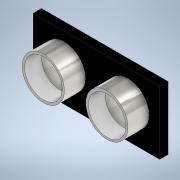
# Autodesk Inventor part: US sensor
Saved by Autodesk Inventor 2021 (Build 250183000, 183)
## iProperties
Created: 2021-07-04
Part Number: US sensor
Material: Generic
Document SubType Name: Modeling
Designer: Manojgouda K R
Density: 1 g/cm^3
Appearance: Default
Author: Manojgouda K R
Autodesk Inventor part; units mm, degrees
ref_plane "YZ Plane" through (0, 0, 0) normal (1, 0, 0) x (0, 1, 0)
ref_plane "XZ Plane" through (0, 0, 0) normal (0, 1, 0) x (-1, 0, 0)
ref_plane "XY Plane" through (0, 0, 0) normal (0, 0, 1) x (1, 0, 0)
sketch "Sketch1" plane through (0, 0, 0) normal (0, 0, 1) x (1, 0, 0)
  line L0 (-9.2175, -0.9972) -> (-3.2175, -0.9972)
  line L1 (-3.2175, -0.9972) -> (-3.2175, -3.9972)
  line L2 (-3.2175, -3.9972) -> (-9.2175, -3.9972)
  line L3 (-9.2175, -3.9972) -> (-9.2175, -0.9972)
  point P0 (0, 0)
  dimension "d0" = 6
  dimension "d1" = 3
  dimension "d2" = 6
  constraints: 8 end point, 2 parallel, 1 horizontal, 1 perpendicular
  measures "d0" distance of L1.end L2.end
  measures "d1" distance of L0.end L1.end
  measures "d2" distance of L0.start L0.end
extrude "Extrusion1" add sketch "Sketch1" along normal blind 0.4
sketch "Sketch2" plane through (0, 0, 0.4) normal (0, 0, 1) x (1, 0, 0)
  circle A0 centre (-7.7322, -2.4245) radius 1
  circle A1 centre (-4.718, -2.4245) radius 1
  point P0 (0, 0)
  dimension "d5" = 2
  dimension "d6" = 2
  constraints: 2 centre point
  measures "d5" diameter of A0
  measures "d6" diameter of A1
extrude "Extrusion2" add sketch "Sketch2" along normal blind 1
sketch "Sketch3" plane through (-7.7322, -2.4245, 1.4) normal (0, 0, 1) x (1, 0, 0)
  point P0 (7.7322, 2.4245)
  point P1 (0.0073, 0.0096)
  point P2 (3.0276, -0.0199)
hole "Hole1" at (-7.7249, -2.4149, 1.4) at (-4.7046, -2.4445, 1.4) direction (0, 0, -1) diameter 1.778 depth 0.8 tip angle 118 clearance for "Flat Head Machine Screw (82)" size "#0" standard "Ansi Unified Screw Threads"
body "Solid1"
